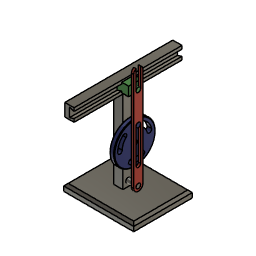
assamble (Autodesk Fusion 360 design; units mm, degrees)
Autodesk Fusion 360 part; units mm, degrees
sketch "Sketch1" plane through (0, 0, 0) normal (0, 1, 0) x (1, 0, 0)
  line L0 (61, 6) -> (-61, 6)
  line L1 (-61, 6) -> (-61, -6)
  line L2 (-61, -6) -> (61, -6)
  line L3 (61, -6) -> (61, 6)
  line L4 (61, 6) -> (-61, -6) construction
  line L5 (-61, 6) -> (61, -6) construction
  line L6 (-16, -172) -> (0, -172)
  line L7 (0, -172) -> (0, -6)
  line L8 (0, -6) -> (-16, -6)
  line L9 (-16, -6) -> (-16, -172)
  line L10 (0, -20) -> (18, -20)
  line L11 (18, -20) -> (18, -16)
  line L12 (18, -16) -> (0, -16)
  line L13 (0, -16) -> (0, -20)
  line L14 (0, -82) -> (12, -82)
  line L15 (12, -82) -> (12, -78)
  line L16 (12, -78) -> (0, -78)
  line L17 (0, -78) -> (0, -82)
  line L18 (0, -169) -> (12, -169)
  line L19 (12, -169) -> (12, -153)
  line L20 (12, -153) -> (0, -153)
  line L21 (0, -153) -> (0, -169)
  line L22 (12, -161) -> (18, -161)
  line L23 (18, -161) -> (18, -165)
  line L24 (18, -165) -> (12, -165)
  line L25 (12, -165) -> (12, -161)
  line L26 (0, -161) -> (-8, -161) construction
  line L27 (-8, -161) -> (-8, -169)
  line L28 (-8, -169) -> (0, -166.4006)
  line L29 (-8, -161) -> (-8, -153)
  line L30 (-8, -153) -> (0, -155.5994)
  line L31 (-16, -150) -> (0, -150)
  line L32 (4, -114) -> (12, -114)
  line L33 (12, -114) -> (12, -82)
  line L34 (12, -82) -> (4, -82)
  line L35 (4, -82) -> (4, -114)
  line L36 (12, -112) -> (18, -112)
  line L37 (18, -112) -> (18, -108)
  line L38 (18, -108) -> (12, -108)
  line L39 (12, -108) -> (12, -112)
  dimension "d31" = 122
  dimension "d32" = 12
  dimension "d33" = 166
  dimension "d34" = 16
  dimension "d35" = 10
  dimension "d36" = 4
  dimension "d37" = 72
  dimension "d38" = 4
  dimension "d39" = 3
  dimension "d40" = 16
  dimension "d41" = 12
  dimension "d42" = 6
  dimension "d43" = 4
  dimension "d44" = 8
  dimension "d45" = 8
  dimension "d46" = 18
  dimension "d47" = -22
  dimension "d48" = 32
  dimension "d49" = 8
  dimension "d50" = 2
  dimension "d51" = 4
  constraint horizontal L0
  constraint perpendicular L0 L1
  constraint parallel L0 L2
  constraint parallel L1 L3
  constraint coincident L4 origin
  constraint coincident L5 origin
  constraint horizontal L6
  constraint vertical L7
  constraint horizontal L8
  constraint vertical L9
  constraint midpoint L2 L7.end
  constraint horizontal L10
  constraint vertical L11
  constraint horizontal L12
  constraint vertical L13
  constraint coincident L7 L10.start
  constraint horizontal L14
  constraint vertical L15
  constraint horizontal L16
  constraint vertical L17
  constraint coincident L7 L14.start
  constraint horizontal L18
  constraint vertical L19
  constraint horizontal L20
  constraint vertical L21
  constraint coincident L7 L18.start
  constraint horizontal L22
  constraint vertical L23
  constraint horizontal L24
  constraint vertical L25
  constraint midpoint L19 L22.start
  constraint midpoint L21 L26.start
  constraint perpendicular L21 L26
  constraint perpendicular L26 L27
  constraint coincident L7 L28.end
  constraint symmetric L27.start L26 L29.start
  constraint symmetric L26 L27.end L29.end
  constraint symmetric L26 L28.end L30.end
  constraint horizontal L32
  constraint vertical L33
  constraint horizontal L34
  constraint vertical L35
  constraint horizontal L36
  constraint vertical L37
  constraint horizontal L38
  constraint vertical L39
  constraint coincident L33 L36.start
  constraint vertical L22.end L36.end
  constraint vertical L19.end L32.end
  constraint vertical L10.end L37.end
  measures "d31" distance of L1.end L2.end
  measures "d32" distance of L0.end L1.end
  measures "d33" distance of L6.start L8.end
  measures "d34" distance of L6.start L6.end
  measures "d35" distance of L7.end L12
  measures "d36" distance of L10.end L11.end
  measures "d37" distance of L2 L15.end
  measures "d38" distance of L14.end L15.end
  measures "d39" distance of L6.end L18
  measures "d40" distance of L18.end L19.end
  measures "d41" distance of L18.start L18.end
  measures "d42" distance of L22.start L22.end
  measures "d43" distance of L22.end L23.end
  measures "d44" distance of L26.start L26.end
  measures "d45" distance of L26.end L27.end
  measures "d46" angle of L18 L28
  measures "d48" distance of L32.start L34.end
  measures "d49" distance of L32.start L32.end
  measures "d50" distance of L32.end L36
  measures "d51" distance of L36.end L37.end
extrude "Extrude1" add sketch "Sketch1" along normal mid plane 102 contours L0 L1 L2 L3 L8 makes body 1
extrude "Extrude2" add sketch "Sketch1" along normal mid plane 18 contours L2 L7 L8 L9 L13 L17 L31 bodies 1
extrude "Extrude3" add sketch "Sketch1" along normal mid plane 188 contours L6 L7 L9 L21 L27 L28 L29 L30 L31 bodies 1
extrude "Extrude4" add sketch "Sketch1" along normal mid plane 22 separate body contours L7 L18 L19 L20 L21 L25 | L7 L21 L27 L28 L29 L30 makes body 2
revolve "Revolve1" add sketch "Sketch1" angle 360 about axis through (12, 0, 161) along (1, 0, 0) contours L19 L22 L23 L24 L25 bodies 2
revolve "Revolve2" add sketch "Sketch1" angle 360 about axis through (12, 0, 78) along (-1, 0, 0) contours L7 L14 L15 L16 L17 L34 bodies 1
revolve "Revolve3" add sketch "Sketch1" angle 360 about axis through (12, 0, 78) along (-1, 0, 0) separate body contours L14 L32 L33 L34 L35 L39 makes body 3
revolve "Revolve4" add sketch "Sketch1" angle 360 about axis through (18, 0, 108) along (-1, 0, 0) contours L33 L36 L37 L38 L39 bodies 3
revolve "Revolve5" add sketch "Sketch1" angle 360 about axis through (18, 0, 16) along (-1, 0, 0) contours L7 L10 L11 L12 L13 bodies 1
sketch "Sketch2" plane through (12, 0, 0) normal (1, 0, 0) x (0, 1, 0)
  circle A0 centre (0, 108) radius 4
  circle A1 centre (0, 78) radius 4
  circle A2 centre (0, 78) radius 36
  arc A3 (-20.8398, 99.5802) -> (-30, 78) centre (0, 78) ccw
  arc A4 (-15.2825, 93.8255) -> (-20.8398, 99.5802) centre (-18.0611, 96.7028) ccw
  arc A5 (-15.2825, 93.8255) -> (-22, 78) centre (0, 78) ccw
  arc A6 (-30, 78) -> (-22, 78) centre (-26, 78) ccw
  arc A7 (-18.0611, 96.7028) -> (-26, 78) centre (0, 78) ccw construction
  point P0 (0, 78)
  dimension "d65" = 26
  dimension "d66" = 4
  dimension "d67" = 46
  constraint tangent A3 A4
  constraint tangent A4 A5
  constraint tangent A5 A6
  constraint tangent A3 A6
  constraint coincident P0 A1.centre
  constraint horizontal A6.centre P0
  measures "d65" radius of A7
  measures "d66" radius of A4
  measures "d67" angle of A6.centre A4.centre P0
extrude "Extrude5" cut sketch "Sketch2" against normal up to surface (8 mm away) contours A3 A4 A5 A6 bodies 3
pattern_circular "C-Pattern1" count 3 over 360 about axis through (12, 0, 78) along (-1, 0, 0) of "Extrude5"
sketch "Sketch3" plane through (18, 0, 0) normal (1, 0, 0) x (0, 1, 0)
  circle A0 centre (0, 16) radius 4
  line L0 (8, 16) -> (8, 188)
  arc A1 (8, 188) -> (-8, 188) centre (0, 188) ccw
  line L1 (-8, 188) -> (-8, 16)
  arc A2 (-8, 16) -> (8, 16) centre (0, 16) ccw
  line L2 (0, 16) -> (0, 188) construction
  circle A3 centre (0, 161) radius 4
  circle A4 centre (0, 108) radius 4
  circle A5 centre (0, 78) radius 4
  circle A6 centre (0, 16) radius 4
  line L3 (4, 161) -> (4, 196)
  arc A7 (4, 196) -> (-4, 196) centre (0, 196) ccw
  line L4 (-4, 196) -> (-4, 161)
  arc A8 (-4, 161) -> (4, 161) centre (0, 161) ccw
  line L5 (0, 161) -> (0, 196) construction
  line L6 (-4, 108) -> (-4, 48)
  arc A9 (-4, 48) -> (4, 48) centre (0, 48) ccw
  line L7 (4, 48) -> (4, 108)
  arc A10 (4, 108) -> (-4, 108) centre (0, 108) ccw
  line L8 (0, 108) -> (0, 48) construction
  dimension "d72" = 172
  dimension "d73" = 8
  dimension "d74" = 60
  constraint tangent L0 A1
  constraint tangent A1 L1
  constraint parallel L0 L1
  constraint tangent L1 A2
  constraint tangent L0 A2
  constraint vertical L2
  constraint coincident A0.centre A2.centre
  constraint tangent L3 A7
  constraint tangent A7 L4
  constraint parallel L3 L4
  constraint tangent L4 A8
  constraint tangent L3 A8
  constraint parallel L2 L5
  constraint coincident A3.centre A8.centre
  constraint equal A3 A8
  constraint coincident A1 A7.centre
  constraint tangent L6 A9
  constraint tangent A9 L7
  constraint parallel L6 L7
  constraint tangent L7 A10
  constraint tangent L6 A10
  constraint parallel L2 L8
  constraint coincident A4.centre A10.centre
  constraint equal A4 A10
  measures "d72" distance of A0.centre A1.centre
  measures "d73" radius of A1
  measures "d74" distance of A4.centre A9.centre
extrude "Extrude6" add sketch "Sketch3" against normal blind 4 separate body contours L0 A1 L1 A2 A3 L3 L4 A8 makes body 4
chamfer "Chamfer1" distance 1 angle 45 2 edges at (12, -13.0182, 44.4362) (4, -13.0182, 44.4362) on bodies 3
chamfer "Chamfer2" distance 4 angle 45 4 edges at (-61, 0, 6) (0, -51, 6) (61, 0, 6) (0, 51, 6) on bodies 1
copy_body "Body->Comp1" bodies 2 removing the originals makes body 5 in component "slider"
copy_body "Body->Comp2" bodies 3 removing the originals makes body 6 in component "disk"
copy_body "Body->Comp3" bodies 4 removing the originals makes body 7 in component "crank"
copy_body "Body->Comp4" bodies 1 removing the originals makes body 8 in component "base"
component "disk" placed x (1, 0, 0) y (0, 1, 0) z (0, 0, 1) at (0, 0, 0)
component "crank" placed x (1, 0, 0) y (0, 1, 0) z (0, 0, 1) at (0, 0, 0)
component "slider" placed x (1, 0, 0) y (0, 1, 0) z (0, 0, 1) at (0, 0, 0)
component "base" placed x (1, 0, 0) y (0, 1, 0) z (0, 0, 1) at (0, 0, 0)
